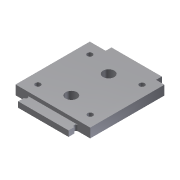
# Autodesk Inventor part: JointC0_
Saved by Autodesk Inventor 2013 (Build 170138000, 138)
## iProperties
Created: 2012-12-03
Part Number: JointC0_
Document SubType Name: Modeling
Designer: JohnHenry
Density: 1 g/cm^3
Material: 一般
Mass: 8.36147 g
Surface Area: 47.972 cm^2
Volume: 8.36147 cm^3
Author: JohnHenry
Autodesk Inventor part; units mm, degrees
ref_plane "YZ Plane" through (0, 0, 0) normal (1, 0, 0) x (0, 1, 0)
ref_plane "XZ Plane" through (0, 0, 0) normal (0, 1, 0) x (-1, 0, 0)
ref_plane "XY Plane" through (0, 0, 0) normal (0, 0, 1) x (1, 0, 0)
sketch "スケッチ1" plane through (0, 0, 0) normal (0, 0, 1) x (1, 0, 0)
  line L0 (-20, 25) -> (20, 25)
  line L1 (20, 25) -> (20, -25)
  line L2 (20, -25) -> (-20, -25)
  line L3 (-20, -25) -> (-20, 25)
  point P0 (0, 0)
  dimension "d0" = 50
  dimension "d1" = 40
  dimension "d2" = 20
  dimension "d3" = 25
  constraints: 8 end point, 2 parallel, 1 horizontal, 1 perpendicular
  measures "d0" distance of L2.end L0.start
  measures "d1" distance of L1.end L2.end
  measures "d2" distance from line of L3 point (0, 0)
  measures "d3" distance from line of L2 point (0, 0)
extrude "押し出し1" add sketch "スケッチ1" along normal blind 5
sketch "スケッチ2" plane through (0, 0, 5) normal (0, 0, 1) x (1, 0, 0)
  line L0 (20, 25) -> (20, -25) projected
  line L1 (-20, -25) -> (-20, 25) projected
  line L2 (20, -25) -> (-20, -25) projected
  line L3 (-20, 25) -> (20, 25)
  line L4 (20, 25) -> (20, 19.9)
  line L5 (20, 19.9) -> (-20, 19.9)
  line L6 (-20, 19.9) -> (-20, 25)
  line L7 (20, -25) -> (-20, -25)
  line L8 (-20, -25) -> (-20, -19.9)
  line L9 (-20, -19.9) -> (20, -19.9)
  line L10 (20, -19.9) -> (20, -25)
  point P0 (0, 0)
  dimension "d6" = 5.1
  dimension "d7" = 5.1
  dimension "d12" = 0
  constraints: 16 end point, 4 parallel, 3 point on line, 2 horizontal, 2 perpendicular
  measures "d6" distance between parallel lines of L5 L3
  measures "d7" distance between parallel lines of L2 L9
  measures "d12" distance between parallel lines of L0 L10
extrude "押し出し3" cut sketch "スケッチ2" against normal blind 2 contours L0 L5 L1 L3 | L0 L2 L1 L9
sketch "スケッチ3" plane through (0, 0, 5) normal (0, 0, 1) x (1, 0, 0)
  point P0 (0, 0)
  point P1 (0, 10)
  point P2 (0, -10)
  dimension "d13" = 20
  dimension "d14" = 10
  measures "d13" distance of point (0, -10) point (0, 10)
  measures "d14" distance of point (0, -10) point (0, 0)
hole "Hole1" at (0, 10, 5) at (0, -10, 5) direction (0, 0, -1) diameter 6 end through all
sketch "スケッチ4" plane through (0, 0, 0) normal (0, 0, -1) x (-1, 0, 0)
  circle A0 centre (0, -10) radius 3 projected
  circle A1 centre (0, 10) radius 3 projected
  line L0 (20, 25) -> (-20, 25) projected
  line L1 (-20, 25) -> (-13.5, 25)
  line L2 (-13.5, 25) -> (-13.5, 19.9)
  line L3 (-13.5, 19.9) -> (-20, 19.9)
  line L4 (-20, 19.9) -> (-20, 25)
  line L5 (20, 25) -> (13.5, 25)
  line L6 (13.5, 25) -> (13.5, 19.9)
  line L7 (13.5, 19.9) -> (20, 19.9)
  line L8 (20, 19.9) -> (20, 25)
  line L9 (20, -25) -> (13.5, -25)
  line L10 (13.5, -25) -> (13.5, -19.9)
  line L11 (13.5, -19.9) -> (20, -19.9)
  line L12 (20, -19.9) -> (20, -25)
  line L13 (-20, -25) -> (-13.5, -25)
  line L14 (-13.5, -25) -> (-13.5, -19.9)
  line L15 (-13.5, -19.9) -> (-20, -19.9)
  line L16 (-20, -19.9) -> (-20, -25)
  point P0 (0, 0)
  dimension "d22" = 5.1
  dimension "d23" = 5.1
  dimension "d24" = 5.1
  dimension "d25" = 5.1
  dimension "d26" = 27
  dimension "d27" = 13.5
  dimension "d28" = 13.5
  dimension "d29" = 27
  constraints: 32 end point, 8 parallel, 4 horizontal, 4 perpendicular
  measures "d22" distance of L1.end L2.end
  measures "d23" distance between parallel lines of L7 L0
  measures "d24" distance between parallel lines of L13 L15
  measures "d25" distance of L9.end L10.end
  measures "d26" distance between parallel lines of L6 L2
  measures "d27" distance from line of A1.centre L6
  measures "d28" distance from line of A0.centre L10
  measures "d29" distance between parallel lines of L14 L10
extrude "押し出し4" cut sketch "スケッチ4" against normal through all contours L8 L7 L6 L0 | L2 L3 L4 L0 | L9 L10 L11 L12 | L16 L15 L14 L13
sketch "スケッチ5" plane through (0, 0, 5) normal (0, 0, 1) x (1, 0, 0)
  line L0 (20, 19.9) -> (-20, 19.9) projected
  line L1 (-20, -19.9) -> (-20, 19.9) projected
  line L2 (-20, -19.9) -> (20, -19.9) projected
  line L3 (20, 19.9) -> (20, -19.9) projected
  point P0 (0, 0)
  point P1 (-14, 13.9)
  point P2 (-14, -13.9)
  point P3 (14, -13.9)
  point P4 (14, 13.9)
  dimension "d32" = 6
  dimension "d33" = 6
  dimension "d34" = 6
  dimension "d35" = 6
  dimension "d36" = 6
  dimension "d37" = 6
  dimension "d38" = 6
  dimension "d39" = 6
  measures "d32" distance from line of point (-14, 13.9) L0
  measures "d33" distance from line of L1 point (-14, 13.9)
  measures "d34" distance from line of L2 point (-14, -13.9)
  measures "d35" distance from line of L1 point (-14, -13.9)
  measures "d36" distance from line of point (14, -13.9) L3
  measures "d37" distance from line of L2 point (14, -13.9)
  measures "d38" distance from line of point (14, 13.9) L0
  measures "d39" distance from line of L3 point (14, 13.9)
hole "Hole2" at (-14, 13.9, 5) at (-14, -13.9, 5) at (14, -13.9, 5) at (14, 13.9, 5) direction (0, 0, -1) diameter 2.8 depth 8 tip angle 118
sketch "スケッチ6" plane through (0, 0, 0) normal (0, 0, -1) x (-1, 0, 0)
  line L0 (-20, -19.9) -> (-13.5, -19.9) projected
  line L1 (-13.5, -19.9) -> (-13.5, -25) projected
  line L2 (13.5, -25) -> (13.5, -19.9) projected
  line L3 (13.5, -19.9) -> (20, -19.9) projected
  line L4 (20, 19.9) -> (13.5, 19.9) projected
  line L5 (13.5, 19.9) -> (13.5, 25) projected
  line L6 (-13.5, 19.9) -> (-20, 19.9) projected
  line L7 (-13.5, 19.9) -> (-13.5, 25) projected
  point P0 (0, 0)
  point P1 (-13.5, 20.9)
  point P2 (13.5, 20.9)
  point P3 (13.5, -20.9)
  point P4 (-13.5, -20.9)
  dimension "d47" = 1
  dimension "d48" = 1
  dimension "d49" = 1
  dimension "d50" = 1
  constraints: 4 point on line
  measures "d47" distance from line of L6 point (-13.5, 20.9)
  measures "d48" distance from line of L4 point (13.5, 20.9)
  measures "d49" distance from line of L0 point (-13.5, -20.9)
  measures "d50" distance from line of L3 point (13.5, -20.9)
hole "Hole3" at (13.5, 20.9, 0) at (-13.5, 20.9, 0) at (-13.5, -20.9, 0) at (13.5, -20.9, 0) direction (0, 0, 1) diameter 2 depth 8 tip angle 118
equation "\"d2\" = 0.5 * d1"
equation "\"d3\" = 0.5 * d0"
equation "\"d14\" = 0.5 * d13"
equation "\"d23\" = d22"
equation "\"d24\" = d22"
equation "\"d25\" = d22"
equation "\"d27\" = 0.5 * d26"
equation "\"d28\" = d27"
equation "\"d29\" = d26"
equation "\"d33\" = d32"
equation "\"d34\" = d32"
equation "\"d35\" = d32"
equation "\"d36\" = d32"
equation "\"d37\" = d32"
equation "\"d38\" = d32"
equation "\"d39\" = d32"
equation "\"d48\" = d47"
equation "\"d49\" = d47"
equation "\"d50\" = d47"
